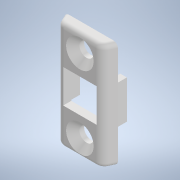
# Autodesk Inventor part: camera_cup
Saved by Autodesk Inventor 2022 (Build 260153000, 153)
## iProperties
Created: 2024-12-22
Part Number: camera_cup
Material: Типовые
Document SubType Name: Modeling
Designer: Andrey
Density: 1 g/cm^3
Appearance: По умолчанию
Author: Andrey
Autodesk Inventor part; units mm, degrees
ref_plane "YZ Plane" through (0, 0, 0) normal (1, 0, 0) x (0, 1, 0)
ref_plane "XZ Plane" through (0, 0, 0) normal (0, 1, 0) x (-1, 0, 0)
sketch "Эскиз1" plane through (0, 0, 0) normal (0, 0, 1) x (1, 0, 0)
  line L0 (-4.25, 4.25) -> (4.25, 4.25) projected
  line L1 (4.25, 4.25) -> (4.25, -4.25) projected
  line L2 (4.25, -4.25) -> (-4.25, -4.25) projected
  line L3 (-4.25, -4.25) -> (-4.25, 4.25) projected
  line L4 (7, -7) -> (7, 7) projected
  line L5 (-7, 7) -> (-7, 4.25) projected
  line L6 (-7, 4.25) -> (-11, 4.25) projected
  line L7 (-11, 4.25) -> (-11, -4.25) projected
  line L8 (-11, -4.25) -> (-7, -4.25) projected
  line L9 (-7, -4.25) -> (-7, -7) projected
  line L10 (-3.75, 3.75) -> (3.75, 3.75)
  line L11 (3.75, 3.75) -> (3.75, -3.75)
  line L12 (3.75, -3.75) -> (-3.75, -3.75)
  line L13 (-3.75, -3.75) -> (-3.75, 3.75)
  line L14 (5.9972, -12) -> (5.9972, -7.2) projected
  line L15 (-5.9972, -7.2) -> (-5.9972, -12) projected
  line L16 (5.9972, -12) -> (-5.9972, -12) projected
  line L17 (5.9972, 7.2) -> (5.9972, 12) projected
  line L18 (-5.9972, 12) -> (5.9972, 12) projected
  line L19 (-5.9972, 12) -> (-5.9972, 7.2) projected
  line L20 (-5.9972, -12) -> (5.9972, -12)
  line L21 (5.9972, -12) -> (5.9972, 12)
  line L22 (5.9972, 12) -> (-5.9972, 12)
  line L23 (-5.9972, 12) -> (-5.9972, -12)
  circle A0 centre (0, -8.25) radius 1.6 projected
  circle A1 centre (0, 8.25) radius 1.6 projected
  point P0 (0, 0)
  dimension "d0" = 0.5
  constraints: 16 end point, 2 parallel, 1 horizontal, 1 perpendicular, 3 other
  measures "d0" distance between parallel lines of L3 L13
extrude "Выдавливание1" add sketch "Эскиз1" along normal blind 0.4 contours L0 L1 L2 L3 | L16 L15 L23 L19 L18 L17 L21 L14
sketch "Эскиз3" plane through (0, 0, 0) normal (0, 0, -1) x (-1, 0, 0)
  line L0 (-5.9972, 12) -> (5.9972, 12) projected
  line L1 (-5.9972, -12) -> (-5.9972, 12) projected
  line L2 (5.9972, -12) -> (-5.9972, -12) projected
  line L3 (5.9972, 12) -> (5.9972, -12) projected
  line L4 (3.75, 3.75) -> (-3.75, 3.75) projected
  line L5 (3.75, -3.75) -> (3.75, 3.75) projected
  line L6 (-3.75, -3.75) -> (3.75, -3.75) projected
  line L7 (-3.75, 3.75) -> (-3.75, -3.75) projected
  line L8 (-4.25, 4.25) -> (4.25, 4.25)
  line L9 (4.25, 4.25) -> (4.25, -4.25)
  line L10 (4.25, -4.25) -> (-4.25, -4.25)
  line L11 (-4.25, -4.25) -> (-4.25, 4.25)
  line L12 (4.5, 4.5) -> (-4.5, 4.5)
  line L13 (-4.5, 4.5) -> (-4.5, -4.5)
  line L14 (-4.5, -4.5) -> (4.5, -4.5)
  line L15 (4.5, -4.5) -> (4.5, 4.5)
  circle A0 centre (0, -8.25) radius 1.6 projected
  circle A1 centre (0, 8.25) radius 1.6 projected
  point P0 (0, 0)
  dimension "d6" = 0.5
  dimension "d7" = 0.25
  constraints: 16 end point, 6 other
  measures "d6" distance between parallel lines of L4 L8
  measures "d7" distance between parallel lines of L8 L12
ref_plane "РабПлоскость2" through (-5.9972, 7.2, -2.1597) normal (0, 0, 1) x (1, 0, 0)
extrude "Выдавливание3" add sketch "Эскиз3" along normal up to surface (2.1597 mm away) contours L0 L3 L2 L1
sketch "Эскиз5" plane through (5.9972, -12, -2.1597) normal (0, 0, -1) x (-1, 0, 0)
  line L0 (-1.6742, 4.8) -> (-1.6742, 19.2) projected
  line L1 (-1.6742, 19.2) -> (13.6686, 19.2) projected
  line L2 (13.6686, 19.2) -> (13.6686, 4.8) projected
  line L3 (13.6686, 4.8) -> (-1.6742, 4.8) projected
  line L4 (13.4686, 19) -> (-1.4742, 19)
  line L5 (-1.4742, 19) -> (-1.4742, 5)
  line L6 (-1.4742, 5) -> (13.4686, 5)
  line L7 (13.4686, 5) -> (13.4686, 19)
  line L8 (1.4972, 16.5) -> (10.4972, 16.5) projected
  line L9 (10.4972, 16.5) -> (10.4972, 7.5) projected
  line L10 (10.4972, 7.5) -> (1.4972, 7.5) projected
  line L11 (1.4972, 7.5) -> (1.4972, 16.5) projected
  line L12 (0, 24) -> (0, 0) projected
  line L13 (0, 0) -> (11.9944, 0) projected
  line L14 (11.9944, 0) -> (11.9944, 24) projected
  line L15 (11.9944, 24) -> (0, 24) projected
  line L16 (0, 7.5) -> (11.9944, 7.5) projected
  line L17 (11.9944, 16.5) -> (0, 16.5) projected
  line L18 (0, 7.7) -> (11.9944, 7.7)
  line L19 (11.9944, 16.3) -> (0, 16.3)
  point P0 (5.9972, 12)
  point P1 (11.9944, 5)
  point P2 (11.9944, 19)
  point P3 (0, 19)
  point P4 (0, 5)
  point P5 (10.4972, 16.3)
  point P6 (10.4972, 7.7)
  point P7 (11.9944, 7.7)
  point P8 (1.4972, 16.3)
  point P9 (0, 16.3)
  point P10 (0, 7.7)
  point P11 (1.4972, 7.7)
  dimension "d13" = 0.2
  dimension "d20" = 0.2
  dimension "d21" = 0.2
  constraints: 12 end point, 2 parallel, 3 other
  measures "d13" distance between parallel lines of L1 L4
  measures "d20" distance between parallel lines of L16 L18
  measures "d21" distance between parallel lines of L17 L19
extrude "Выдавливание5" add sketch "Эскиз5" along normal blind 2 contours L12 L19 L11 L18 | L18 L9 L19 L14
sketch "Эскиз6" plane through (-5.9972, -12, 0.4) normal (0, -1, 0) x (1, 0, 0)
  line L0 (13.5091, -5.808) -> (11.9944, -2.5597) projected
  line L1 (11.9944, -2.5597) -> (0, -2.5597) projected
  line L2 (0, -2.5597) -> (-1.5147, -5.808) projected
  arc A0 (-1.5147, -5.808) -> (13.5091, -5.808) centre (5.9972, 3.55) ccw projected
  line L3 (0, -2.5597) -> (11.9944, -2.5597) projected
  line L4 (0, -2.5597) -> (1.1936, 0)
  line L5 (0, 0) -> (11.9944, 0) projected
  line L6 (11.9944, -2.5597) -> (11.9944, 0) projected
  line L7 (11.9944, -2.5597) -> (10.8008, 0)
  line L8 (13.4686, -2.5597) -> (11.9944, -2.5597) projected
  line L9 (6.996, -2.5597) -> (11.9944, -2.5597) projected
  line L10 (0, -2.5597) -> (-1.4742, -2.5597) projected
  line L11 (-1.4742, -2.5597) -> (-1.4742, -4.5597) projected
  line L12 (13.4686, -4.5597) -> (-1.4742, -4.5597) projected
  line L13 (13.4686, -2.5597) -> (13.4686, -4.5597) projected
  line L14 (11.9944, -2.5597) -> (11.9944, 0) projected
  line L15 (0, 0) -> (11.9944, 0) projected
  line L16 (0, -2.5597) -> (0, 0) projected
  line L17 (11.9944, -2.5597) -> (0, -2.5597) projected
  line L18 (6.996, -2.5597) -> (4.9985, -2.5597) projected
  line L19 (0, -2.5597) -> (4.9985, -2.5597) projected
  point P0 (5.9972, -0.4)
  point P1 (11.9944, -2.5597)
  point P2 (11.9944, -2.5597)
  point P3 (12.927, -4.5597)
  point P4 (-0.9326, -4.5597)
  point P5 (0, -2.5597)
  point P6 (0, -2.5597)
  point P7 (0, -2.5597)
  point P8 (0, -2.5597)
  constraints: 4 end point, 2 collinear, 2 point on line
extrude "Выдавливание6" cut sketch "Эскиз6" against normal up to surface (24 mm away) contours L0 L8 L13 L12 | L7 L5 L6 | L12 L11 L10 L2 | L16 L5 L4
fillet "Сопряжение2" radius 2 2 edges at (-4.8036, 0, 0.4) (4.8036, 0, 0.4)
fillet "Сопряжение3" radius 1 10 edges at (0, -12, 0.4) (4.6041, -12, 0.0868) (5.6696, -12, -1.4572) (-5.6696, -12, -1.4572) (-4.6041, -12, 0.0868) (-5.6696, 12, -1.4572) (0, 12, 0.4) (4.6041, 12, 0.0868) (5.6696, 12, -1.4572) (-4.6041, 12, 0.0868)
chamfer "Фаска1" distance 1.5 angle 45 2 edges at (-1.6, -8.25, 0.4) (-1.6, 8.25, 0.4)
